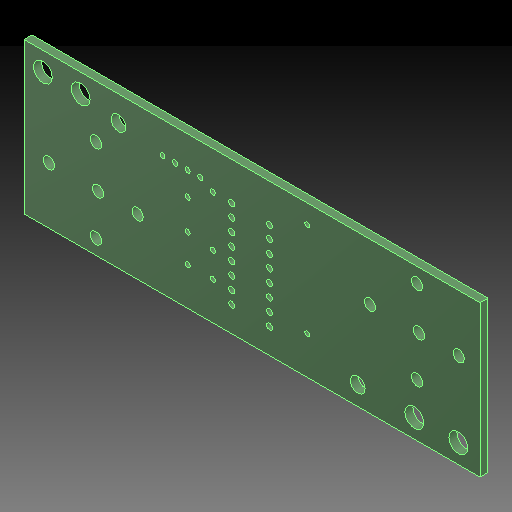
# Autodesk Inventor part: power_pcb.brdКонтур1
Saved by Autodesk Inventor 2020 (Build 240168000, 168)
## iProperties
Created: 2021-08-06
Part Number: power_pcb.brdКонтур1
Material: Типовые
Document SubType Name: Modeling
Designer: Петров Иван
Mass: 4.27884 g
Surface Area: 61.2005 cm^2
Volume: 4.27884 cm^3
Density: 1 g/cm^3
Appearance: Контур панели
Author: Петров Иван
Autodesk Inventor part; units mm, degrees
ref_plane "YZ Plane" through (0, 0, 0) normal (1, 0, 0) x (0, 1, 0)
ref_plane "XZ Plane" through (0, 0, 0) normal (0, 1, 0) x (-1, 0, 0)
ref_plane "XY Plane" through (0, 0, 0) normal (0, 0, 1) x (1, 0, 0)
sketch "Эскиз1" plane through (0, 0, 0) normal (0, 0, 1) x (1, 0, 0)
  line L0 (5.08, 0) -> (97.079, 0)
  line L1 (97.079, 0) -> (97.079, 30.47)
  line L2 (97.079, 30.47) -> (5.08, 30.47)
  line L3 (5.08, 30.47) -> (5.08, 0)
  circle A0 centre (46.99, 22.86) radius 0.6
  circle A1 centre (46.99, 20.32) radius 0.6
  circle A2 centre (46.99, 17.78) radius 0.6
  circle A3 centre (46.99, 15.24) radius 0.6
  circle A4 centre (46.99, 12.7) radius 0.6
  circle A5 centre (46.99, 10.16) radius 0.6
  circle A6 centre (46.99, 7.62) radius 0.6
  circle A7 centre (46.99, 5.08) radius 0.6
  circle A8 centre (54.61, 5.08) radius 0.6
  circle A9 centre (54.61, 7.62) radius 0.6
  circle A10 centre (54.61, 10.16) radius 0.6
  circle A11 centre (54.61, 12.7) radius 0.6
  circle A12 centre (54.61, 15.24) radius 0.6
  circle A13 centre (54.61, 17.78) radius 0.6
  circle A14 centre (54.61, 20.32) radius 0.6
  circle A15 centre (54.61, 22.86) radius 0.6
  circle A16 centre (8.89, 26.67) radius 1.905
  circle A17 centre (92.71, 3.81) radius 1.905
  circle A18 centre (16.51, 26.67) radius 1.905
  circle A19 centre (83.82, 3.81) radius 1.905
  circle A20 centre (33.02, 24.13) radius 0.51
  circle A21 centre (35.56, 24.13) radius 0.51
  circle A22 centre (38.1, 24.13) radius 0.51
  circle A23 centre (40.64, 24.13) radius 0.51
  circle A24 centre (10.1, 11.43) radius 1.15
  circle A25 centre (19.6, 19.83) radius 1.15
  circle A26 centre (19.6, 3.03) radius 1.15
  circle A27 centre (28, 11.43) radius 1.15
  circle A28 centre (20, 11.43) radius 1.15
  circle A29 centre (74.87, 19.05) radius 1.15
  circle A30 centre (84.37, 27.45) radius 1.15
  circle A31 centre (84.37, 10.65) radius 1.15
  circle A32 centre (92.77, 19.05) radius 1.15
  circle A33 centre (84.77, 19.05) radius 1.15
  circle A34 centre (24.13, 25.4) radius 1.5
  circle A35 centre (72.39, 3.81) radius 1.5
  circle A36 centre (43.18, 22.86) radius 0.5
  circle A37 centre (43.18, 12.7) radius 0.5
  circle A38 centre (38.1, 19.431) radius 0.5
  circle A39 centre (38.1, 13.335) radius 0.5
  circle A40 centre (38.1, 7.62) radius 0.5
  circle A41 centre (43.18, 7.62) radius 0.5
  circle A42 centre (62.23, 26.67) radius 0.5
  circle A43 centre (62.23, 7.62) radius 0.5
  constraints: 44 centre point, 8 end point
extrude "power_pcb.brdКонтур" add sketch "Эскиз1" along normal blind 1.6
